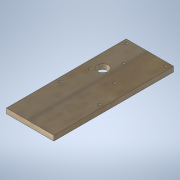
# Autodesk Inventor part: ロボット回転t5.5
Saved by Autodesk Inventor 2020.3 (Build 243373000, 373)
## iProperties
Created: 2020-07-05
Part Number: ロボット回転t5.5
Material: 木材 (カエデ材)
Document SubType Name: Modeling
Designer: totot
Density: 0.67 g/cm^3
Appearance: ナチュラル カエデ材 - 光沢 濃い着色
Mass: 14.9557 g
Surface Area: 101.134 cm^2
Volume: 22.322 cm^3
Author: totot
Autodesk Inventor part; units mm, degrees
ref_plane "YZ Plane" through (0, 0, 0) normal (1, 0, 0) x (0, 1, 0)
ref_plane "XZ Plane" through (0, 0, 0) normal (0, 1, 0) x (-1, 0, 0)
ref_plane "XY Plane" through (0, 0, 0) normal (0, 0, 1) x (1, 0, 0)
sketch "スケッチ1" plane through (0, 0, 0) normal (0, 1, 0) x (-1, 0, 0)
  line L0 (0, 0) -> (-52, 0)
  line L1 (-52, 0) -> (-52, -81.5097)
  line L2 (-52, -81.5097) -> (0, -81.5097)
  line L3 (0, -81.5097) -> (0, 0)
  dimension "d0" = 81.5097
  dimension "d1" = 52
  constraints: 8 end point, 2 parallel, 1 horizontal, 1 perpendicular
  measures "d0" distance between parallel lines of L2 L0
  measures "d1" distance between parallel lines of L1 L3
extrude "押し出し1" add sketch "スケッチ1" along normal blind 5.5
sketch "スケッチ2" plane through (0, 5.5, 0) normal (0, 1, 0) x (1, 0, 0)
  line L0 (0, 0) -> (52, 0) projected
  line L1 (52, 81.5097) -> (0, 81.5097) projected
  line L2 (52, 0) -> (52, 81.5097) projected
  line L3 (0, 81.5097) -> (0, 0) projected
  point P0 (4.5, 4.5)
  point P1 (4.5, 77.0097)
  point P2 (47.5, 77.0097)
  point P3 (47.5, 4.5)
  dimension "d4" = 4.5
  dimension "d5" = 4.5
  dimension "d6" = 4.5
  dimension "d7" = 4.5
  dimension "d8" = 4.5
  dimension "d9" = 4.5
  dimension "d10" = 4.5
  dimension "d11" = 4.5
  measures "d4" distance from line of point (47.5, 4.5) L0
  measures "d5" distance from line of L1 point (47.5, 77.01)
  measures "d6" distance from line of point (47.5, 77.01) L2
  measures "d7" distance from line of L2 point (47.5, 4.5)
  measures "d8" distance from line of L0 point (4.5, 4.5)
  measures "d9" distance from line of L3 point (4.5, 4.5)
  measures "d10" distance from line of L3 point (4.5, 77.01)
  measures "d11" distance from line of L1 point (4.5, 77.01)
hole "穴1" at (4.5, 5.5, -4.5) at (4.5, 5.5, -77.0097) at (47.5, 5.5, -77.0097) at (47.5, 5.5, -4.5) direction (0, -1, 0) diameter 3 end through all
sketch "スケッチ3" plane through (0, 5.5, 0) normal (0, 1, 0) x (1, 0, 0)
  circle A0 centre (22, 40.7548) radius 15.5
  line L0 (0, 0) -> (52, 0) projected
  line L1 (52, 81.5097) -> (0, 81.5097) projected
  line L2 (52, 0) -> (52, 81.5097) projected
  line L3 (22, 40.7548) -> (35.4234, 33.0048)
  line L4 (22, 40.7548) -> (37.5, 40.7548) construction
  line L5 (22, 40.7548) -> (8.5766, 33.0048)
  line L6 (22, 40.7548) -> (22, 56.2548)
  line L7 (22, 40.7548) -> (37.5, 40.7548) construction
  point P0 (4.5, 0)
  point P1 (47.5, 0)
  point P2 (47.5, 81.5097)
  point P3 (4.5, 81.5097)
  point P4 (52, 4.5)
  point P5 (52, 77.0097)
  dimension "d20" = 31
  dimension "d21" = 81.5097
  dimension "d22" = 40.7548
  dimension "d23" = 30
  dimension "d25" = 90
  dimension "d43" = 120
  dimension "d44" = 120
  constraints: 10 end point, 3 coincident, 3 point on circle, 2 equal length, 2 horizontal, 1 centre point
  measures "d20" diameter of A0
  measures "d21" distance between parallel lines of L0 L1
  measures "d22" distance from line of L3.start L1
  measures "d23" distance from line of L3.start L2
  measures "d25" angle of L7 L6
  measures "d43" angle of L6 L5
  measures "d44" angle of L3 L5
hole "穴2" at (35.4234, 5.5, -33.0048) at (22, 5.5, -56.2548) at (8.5766, 5.5, -33.0048) direction (0, -1, 0) diameter 3 end through all
sketch "スケッチ4" plane through (0, 5.5, 0) normal (0, 1, 0) x (1, 0, 0)
  line L0 (0, 0) -> (52, 0) projected
  line L1 (52, 81.5097) -> (0, 81.5097) projected
  line L2 (52, 0) -> (52, 81.5097) projected
  point P0 (15, 40.7548)
  point P1 (4.5, 0)
  point P2 (47.5, 0)
  point P3 (47.5, 81.5097)
  point P4 (4.5, 81.5097)
  point P5 (52, 4.5)
  point P6 (52, 77.0097)
  dimension "d33" = 81.5097
  dimension "d34" = 40.7548
  dimension "d35" = 37
  measures "d33" distance between parallel lines of L0 L1
  measures "d34" distance from line of point (15, 40.755) L1
  measures "d35" distance from line of point (15, 40.755) L2
hole "穴3" at (15, 5.5, -40.7548) direction (0, -1, 0) diameter 12 end through all
sketch "スケッチ5" plane through (0, 0, 0) normal (0, 0, 1) x (1, 0, 0)
  line L0 (0, 0) -> (0, 5.5) projected
  line L1 (52, 0) -> (52, 5.5) projected
  line L2 (0, 0) -> (52, 0)
  line L3 (52, 0) -> (52, 5.5)
  line L4 (52, 5.5) -> (0, 5.5)
  line L5 (0, 5.5) -> (0, 0)
  constraints: 8 end point, 2 parallel, 1 horizontal, 1 perpendicular
extrude "押し出し2" add sketch "スケッチ5" along normal blind 50
sketch "スケッチ6" plane through (0, 5.5, 0) normal (0, 1, 0) x (1, 0, 0)
  line L0 (0, 81.5097) -> (0, -50) projected
  circle A0 centre (15, 40.7548) radius 6 projected
  line L1 (52, -50) -> (0, -50) projected
  point P0 (0, 0)
  point P1 (15, -45.5)
  point P2 (15, -13.07)
  dimension "d47" = 15
  dimension "d48" = 15
  dimension "d49" = 15
  dimension "d57" = 32.43
  dimension "d58" = 4.5
  measures "d47" distance from line of L0 A0.centre
  measures "d48" distance from line of point (15, -13.07) L0
  measures "d49" distance from line of point (15, -45.5) L0
  measures "d57" distance of point (15, -13.07) point (15, -45.5)
  measures "d58" distance from line of point (15, -45.5) L1
hole "穴4" at (15, 5.5, 45.5) at (15, 5.5, 13.07) direction (0, -1, 0) diameter 3 end through all
sketch "スケッチ7" plane through (0, 5.5, 0) normal (0, 1, 0) x (1, 0, 0)
  circle A0 centre (15, -13.07) radius 1.5 projected
  circle A1 centre (15, -45.5) radius 1.5 projected
  line L0 (0, 81.5097) -> (0, -50) projected
  point P0 (0, 0)
  point P1 (15, -29.285)
  dimension "d59" = 32.43
  dimension "d60" = 15
  dimension "d61" = 15
  dimension "d62" = 16.215
  measures "d59" distance of A0.centre A1.centre
  measures "d60" distance from line of A1.centre L0
  measures "d61" distance from line of point (15, -29.285) L0
  measures "d62" distance of point (15, -29.285) A1.centre
hole "穴5" at (15, 5.5, 29.285) direction (0, -1, 0) diameter 8 end through all
fillet "フィレット2" radius 4.5 4 edges at (52, 2.75, 50) (0, 2.75, 50) (52, 2.75, -81.5097) (0, 2.75, -81.5097)
equation "\"d6\" = d5"
equation "\"d7\" = d4"
equation "\"d22\" = 0.5 * d21"
equation "\"d44\" = d43"
equation "\"d34\" = 0.5 * d33"
equation "\"d48\" = d47"
equation "\"d49\" = d48"
equation "\"d61\" = d60"
equation "\"d62\" = 0.5 * d59"
